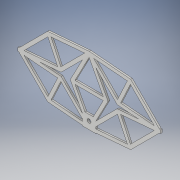
# Autodesk Inventor part: Eye Truss 2
Saved by Autodesk Inventor 2018 (Build 220112000, 112)
## iProperties
Created: 2019-01-14
Part Number: Eye Truss 2
Material: Generic
Document SubType Name: Modeling
Designer: 871357
Density: 1 g/cm^3
Appearance: Default
Author: 871357
Autodesk Inventor part; units mm, degrees
ref_plane "YZ Plane" through (0, 0, 0) normal (1, 0, 0) x (0, 1, 0)
ref_plane "XZ Plane" through (0, 0, 0) normal (0, 1, 0) x (-1, 0, 0)
ref_plane "XY Plane" through (0, 0, 0) normal (0, 0, 1) x (1, 0, 0)
sketch "Sketch1" plane through (0, 0, 0) normal (0, 0, 1) x (1, 0, 0)
  line L0 (0, 0) -> (266.7, 0) construction
  line L1 (266.7, 0) -> (266.7, 127) construction
  line L2 (266.7, 127) -> (0, 127) construction
  line L3 (0, 127) -> (0, 0) construction
  line L4 (3.175, 63.5) -> (57.1495, 117.4745) construction
  line L5 (3.175, 63.5) -> (61.6477, 63.5) construction
  line L6 (133.35, 123.825) -> (209.5505, 117.4745) construction
  line L7 (133.35, 123.825) -> (154.8013, 123.825) construction
  line L8 (133.35, 123.825) -> (57.1495, 117.4745) construction
  line L9 (133.35, 123.825) -> (241.0197, 123.825) construction
  line L10 (133.35, 123.825) -> (79.3755, 69.8505) construction
  line L11 (3.175, 63.5) -> (79.3755, 69.8505) construction
  line L12 (3.175, 63.5) -> (58.3803, 63.5) construction
  line L13 (57.1495, 117.4745) -> (79.3755, 69.8505) construction
  line L14 (263.525, 63.5) -> (334.0804, 63.5) construction
  line L15 (263.525, 63.5) -> (356.1825, 63.5) construction
  line L16 (263.525, 63.5) -> (209.5505, 117.4745) construction
  line L17 (133.35, 123.825) -> (187.3245, 69.8505) construction
  line L18 (263.525, 63.5) -> (187.3245, 69.8505) construction
  line L19 (263.525, 63.5) -> (382.9611, 63.5) construction
  line L20 (187.3245, 69.8505) -> (209.5505, 117.4745) construction
  line L21 (101.6, 63.5) -> (165.1, 63.5) construction
  line L22 (133.35, 123.825) -> (101.6, 63.5) construction
  line L23 (165.1, 63.5) -> (133.35, 123.825) construction
  line L24 (101.6, 63.5) -> (133.35, 3.175) construction
  line L25 (133.35, 3.175) -> (165.1, 63.5) construction
  line L26 (133.35, 3.175) -> (205.0345, 3.175) construction
  line L27 (133.35, 3.175) -> (233.6369, 3.175) construction
  line L28 (133.35, 3.175) -> (200.2999, 3.175) construction
  line L29 (3.175, 63.5) -> (15.875, 63.5) construction
  line L30 (133.35, 3.175) -> (133.35, 50.0944) construction
  line L31 (263.525, 63.5) -> (250.825, 63.5) construction
  line L32 (120.65, 0) -> (146.05, 0)
  circle A0 centre (133.35, 14.1798) radius 3.5449
  line L33 (0, 60.325) -> (1.8599, 60.325)
  line L34 (11.549, 67.3839) -> (56.1894, 112.0242)
  line L35 (56.1894, 112.0242) -> (74.5717, 72.6362)
  line L36 (74.5717, 72.6362) -> (11.549, 67.3839)
  line L37 (61.9533, 114.6888) -> (124.976, 119.9411)
  line L38 (124.976, 119.9411) -> (80.3356, 75.3008)
  line L39 (80.3356, 75.3008) -> (61.9533, 114.6888)
  line L40 (133.35, 127) -> (55.7148, 120.5299)
  line L41 (0, 66.675) -> (1.8599, 66.675)
  line L42 (1.8599, 66.675) -> (55.7148, 120.5299)
  line L43 (0, 66.675) -> (0, 60.325)
  line L44 (120.65, 0) -> (120.65, 1.0584)
  line L45 (120.65, 11.3849) -> (120.65, 7.5306)
  line L46 (106.859, 60.325) -> (125.5486, 24.8146)
  line L47 (106.859, 66.675) -> (133.35, 117.008)
  line L48 (125.5486, 24.8146) -> (141.1514, 24.8146)
  line L49 (106.859, 60.325) -> (133.35, 60.325)
  line L50 (106.859, 66.675) -> (133.35, 66.675)
  line L51 (266.7, 60.325) -> (264.8401, 60.325)
  line L52 (255.151, 67.3839) -> (210.5106, 112.0242)
  line L53 (210.5106, 112.0242) -> (192.1283, 72.6362)
  line L54 (192.1283, 72.6362) -> (255.151, 67.3839)
  line L55 (204.7467, 114.6888) -> (141.724, 119.9411)
  line L56 (141.724, 119.9411) -> (186.3644, 75.3008)
  line L57 (186.3644, 75.3008) -> (204.7467, 114.6888)
  line L58 (133.35, 127) -> (210.9852, 120.5299)
  line L59 (266.7, 66.675) -> (264.8401, 66.675)
  line L60 (264.8401, 66.675) -> (210.9852, 120.5299)
  line L61 (159.841, 60.325) -> (141.1514, 24.8146)
  line L62 (159.841, 66.675) -> (133.35, 117.008)
  line L63 (159.841, 60.325) -> (133.35, 60.325)
  line L64 (159.841, 66.675) -> (133.35, 66.675)
  line L65 (266.7, 66.675) -> (266.7, 60.325)
  line L66 (146.05, 11.3849) -> (146.05, 7.5306)
  line L67 (146.05, 1.0584) -> (146.05, 0)
  line L68 (11.549, 59.6161) -> (56.1894, 14.9758)
  line L69 (56.1894, 14.9758) -> (74.5717, 54.3638)
  line L70 (74.5717, 54.3638) -> (11.549, 59.6161)
  line L71 (61.9533, 12.3112) -> (120.65, 7.4194)
  line L72 (120.65, 11.3849) -> (80.3356, 51.6992)
  line L73 (80.3356, 51.6992) -> (61.9533, 12.3112)
  line L74 (120.65, 1.0584) -> (55.7148, 6.4701)
  line L75 (1.8599, 60.325) -> (55.7148, 6.4701)
  line L76 (264.8401, 60.325) -> (210.9852, 6.4701)
  line L77 (192.1283, 54.3638) -> (255.151, 59.6161)
  line L78 (255.151, 59.6161) -> (210.5106, 14.9758)
  line L79 (210.5106, 14.9758) -> (192.1283, 54.3638)
  line L80 (186.3644, 51.6992) -> (204.7467, 12.3112)
  line L81 (204.7467, 12.3112) -> (146.05, 7.4194)
  line L82 (146.05, 1.0584) -> (210.9852, 6.4701)
  line L83 (146.05, 11.3849) -> (186.3644, 51.6992)
  line L84 (120.65, 7.5306) -> (120.65, 7.4194)
  line L85 (146.05, 7.5306) -> (146.05, 7.4194)
  line L86 (41.4042, 63.5) -> (80.7982, 66.7831)
  line L87 (80.7982, 66.7831) -> (120.7865, 106.7714)
  line L88 (120.7865, 106.7714) -> (98.0121, 63.5)
  line L89 (98.0121, 63.5) -> (120.7865, 20.2286)
  line L90 (120.7865, 20.2286) -> (80.7982, 60.2169)
  line L91 (80.7982, 60.2169) -> (41.4042, 63.5)
  line L92 (225.2958, 63.5) -> (185.9018, 66.7831)
  line L93 (185.9018, 66.7831) -> (145.9135, 106.7714)
  line L94 (145.9135, 106.7714) -> (168.6879, 63.5)
  line L95 (168.6879, 63.5) -> (145.9135, 20.2286)
  line L96 (145.9135, 20.2286) -> (185.9018, 60.2169)
  line L97 (185.9018, 60.2169) -> (225.2958, 63.5)
  point P0 (252.2019, 60.325)
  point P1 (124.976, 7.0589)
  point P2 (133.35, 0)
  point P3 (141.724, 7.0589)
  dimension "d1" = 266.7
  dimension "d2" = 127
  dimension "d4" = 45
  dimension "d6" = 4.764
  dimension "d7" = 175.236
  dimension "d9" = 4.764
  dimension "d10" = 63.5
  dimension "d11" = 133.35
  dimension "d12" = 3.175
  dimension "d13" = 135
  dimension "d14" = 3.175
  dimension "d17" = 3.175
  dimension "d18" = 63.5
  dimension "d19" = 175.236
  dimension "d20" = 45
  dimension "d21" = 45
  dimension "d22" = 31.75
  dimension "d23" = 31.75
  dimension "d24" = 60.325
  dimension "d25" = 133.35
  dimension "d26" = 3.175
  dimension "d32" = 12.7
  dimension "d33" = 120.65
  dimension "d34" = 25.4
  dimension "d37" = 14.1798
  dimension "d38" = 7.0899
  dimension "d46" = 3.175
  dimension "d47" = 3.175
  dimension "d48" = 3.175
  dimension "d49" = 3.175
  dimension "d50" = 3.175
  dimension "d55" = 6.35
  dimension "d56" = 6.35
  dimension "d57" = 3.175
  dimension "d76" = 3.175
  dimension "d77" = 26.4911
  dimension "d78" = 6.35
  dimension "d83" = 4.764
  dimension "d84" = 4.764
  dimension "d85" = 45
  dimension "d86" = 4.764
  dimension "d87" = 4.764
  dimension "d88" = 62.242
  dimension "d89" = 24.8146
  dimension "d90" = 3.8542
  dimension "d91" = 25.4
  dimension "d92" = 1.0584
  dimension "d95" = 6.35
  dimension "d96" = 6.35
  dimension "d97" = 3.175
  dimension "d98" = 3.175
  dimension "d99" = 6.35
  dimension "d100" = 6.35
  dimension "d101" = 45
  dimension "d102" = 6.35
  dimension "d103" = 6.35
  constraints: 196 end point, 38 symmetric about line, 18 parallel, 16 horizontal, 7 point on line, 3 perpendicular, 3 vertical, 2 collinear, 1 centre point, 1 midpoint
  measures "d1" distance of L2.end L1.end
  measures "d2" distance of L1.end L0.end
  measures "d4" angle of L5 L4
  measures "d6" angle of L6 L7
  measures "d7" angle of L8 L9
  measures "d9" angle of L12 L11
  measures "d10" vertical distance of L2.end L4.start
  measures "d11" horizontal distance of L6.start L2.end
  measures "d12" distance from line of L2 L6.start
  measures "d13" angle of L9 L10
  measures "d14" horizontal distance of L4.start L2.end
  measures "d17" distance from line of L1 L14.start
  measures "d18" distance from line of L2 L14.start
  measures "d19" angle of L19 L18
  measures "d20" angle of L9 L17
  measures "d21" angle of L9 L16
  measures "d22" horizontal distance of L6.start L21.end
  measures "d23" horizontal distance of L6.start L21.start
  measures "d24" distance from line of L21 L6.start
  measures "d25" horizontal distance of L0.start L24.end
  measures "d26" distance from line of L0 L24.end
  measures "d32" distance of L4.start L29.end
  measures "d33" distance from line of L1 L32.end
  measures "d34" distance of L32.start L32.end
  measures "d37" distance from line of L0 A0.centre
  measures "d38" diameter of A0
  measures "d46" distance between parallel lines of L13 L35
  measures "d47" distance between parallel lines of L11 L36
  measures "d48" distance between parallel lines of L8 L37
  measures "d49" distance between parallel lines of L10 L38
  measures "d50" distance between parallel lines of L13 L39
  measures "d55" distance between parallel lines of L33 L41
  measures "d56" distance between parallel lines of L34 L42
  measures "d57" distance between parallel lines of L4 L42
  measures "d76" distance between parallel lines of L21 L49
  measures "d77" distance of L46.start L49.end
  measures "d78" distance between parallel lines of L49 L50
  measures "d83" angle of L0 L74
  measures "d84" angle of L0 L71
  measures "d85" angle of L0 L83
  measures "d86" angle of L0 L81
  measures "d87" angle of L0 L82
  measures "d88" angle of L64 L62
  measures "d89" distance between parallel lines of L0 L48
  measures "d90" distance of L45.start L45.end
  measures "d91" distance between parallel lines of L66 L45
  measures "d92" distance of L67.start L32.end
  measures "d95" distance between parallel lines of L36 L86
  measures "d96" distance between parallel lines of L38 L87
  measures "d97" distance between parallel lines of L22 L47
  measures "d98" distance between parallel lines of L24 L46
  measures "d99" distance between parallel lines of L46 L89
  measures "d100" distance between parallel lines of L88 L47
  measures "d101" angle of L0 L72
  measures "d102" distance between parallel lines of L72 L90
  measures "d103" distance between parallel lines of L70 L91
extrude "Extrusion3" add sketch "Sketch1" along normal blind 3.175
body "Solid3"
